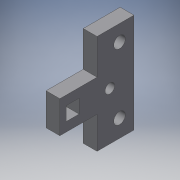
# Autodesk Inventor part: TrayPanelI
Saved by Autodesk Inventor 2017 (Build 210142000, 142)
## iProperties
Created: 2019-06-26
Part Number: TrayPanelI
Material: Generic
Document SubType Name: Modeling
Designer: DDeGo
Density: 1 g/cm^3
Appearance: Default
Author: DDeGo
Autodesk Inventor part; units mm, degrees
ref_plane "YZ Plane" through (0, 0, 0) normal (1, 0, 0) x (0, 1, 0)
ref_plane "XZ Plane" through (0, 0, 0) normal (0, 1, 0) x (-1, 0, 0)
ref_plane "XY Plane" through (0, 0, 0) normal (0, 0, 1) x (1, 0, 0)
sketch "Sketch1" plane through (0, 0, 0) normal (1, 0, 0) x (0, 1, 0)
  line L0 (0, 0) -> (11.5, 0)
  line L1 (11.5, 0) -> (11.5, 31)
  line L2 (11.5, 31) -> (0, 31)
  line L3 (0, 20) -> (-11.6, 20)
  line L4 (-11.6, 20) -> (-11.6, 10)
  line L5 (-11.6, 10) -> (0, 10)
  line L6 (0, 31) -> (0, 20)
  line L7 (0, 10) -> (0, 0)
  line L8 (7, 31) -> (7, 0) construction
  circle A0 centre (7, 26) radius 1.8
  circle A1 centre (7, 5.5) radius 1.8
  line L9 (-11.6, 15) -> (4, 15) construction
  circle A2 centre (4, 15) radius 1.5
  line L10 (-5.6, 12.85) -> (-9.6, 12.85)
  line L11 (-9.6, 12.85) -> (-9.6, 17.15)
  line L12 (-9.6, 17.15) -> (-5.6, 17.15)
  line L13 (-5.6, 17.15) -> (-5.6, 12.85)
  line L14 (-5.6, 12.85) -> (-9.6, 17.15) construction
  line L15 (-9.6, 12.85) -> (-5.6, 17.15) construction
  point P0 (-7.6, 15)
  dimension "d0" = 10
  dimension "d4" = 11.5
  dimension "d7" = 20.5
  dimension "d8" = 3.6
  dimension "d10" = 7
  dimension "d11" = 3
  dimension "d12" = 4
  dimension "d13" = 9.5
  dimension "d14" = 16
  dimension "d15" = 15
  dimension "d16" = 5.6
  dimension "d17" = 4
  dimension "d18" = 4.3
  dimension "d19" = 2
  constraints: 32 end point, 6 parallel, 5 point on line, 4 horizontal, 4 perpendicular, 3 centre point, 3 midpoint, 1 coincident, 1 collinear, 1 equal radius
  measures "d0" distance of L3.end L4.end
  measures "d4" distance of L0.start L0.end
  measures "d7" distance of A0.centre A1.centre
  measures "d8" diameter of A0
  measures "d10" distance between parallel lines of L7 L8
  measures "d11" diameter of A2
  measures "d12" distance from line of L7 A2.centre
  measures "d13" distance from line of L9 A1.centre
  measures "d14" distance between parallel lines of L2 L9
  measures "d15" distance between parallel lines of L0 L9
  measures "d16" distance between parallel lines of L6 L13
  measures "d17" distance between parallel lines of L11 L13
  measures "d18" distance of L10.end L11.end
  measures "d19" distance between parallel lines of L4 L11
extrude "Extrusion1" add sketch "Sketch1" along normal blind 4.3
body "Solid1"
